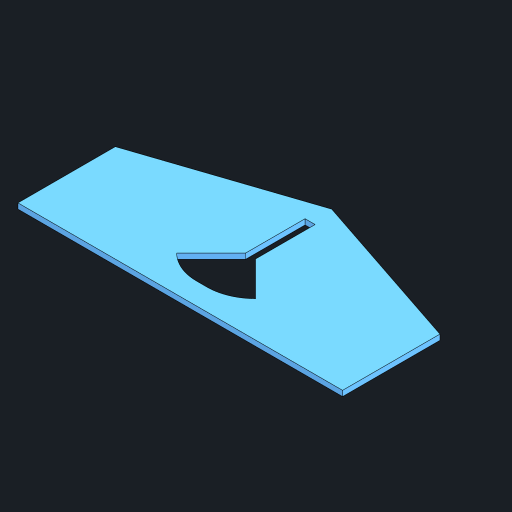
# Autodesk Inventor part: HoriWing
Saved by Autodesk Inventor 2023 (Build 270158000, 158)
## iProperties
Created: 2022-06-06
Part Number: HoriWing
Material: スタイロフォームIB
Document SubType Name: Modeling
Designer: neko2
Density: 0.027 g/cm^3
Appearance: スタイロフォームIB
Mass: 3.48774 g
Surface Area: 570.074 cm^2
Volume: 129.176 cm^3
Author: neko2
Autodesk Inventor part; units mm, degrees
ref_plane "YZ Plane" through (0, 0, 0) normal (1, 0, 0) x (0, 1, 0)
ref_plane "XZ Plane" through (0, 0, 0) normal (0, 1, 0) x (-1, 0, 0)
ref_plane "XY Plane" through (0, 0, 0) normal (0, 0, 1) x (1, 0, 0)
sketch "スケッチ1" plane through (0, 0, 0) normal (0, 1, 0) x (-1, 0, 0)
  line L0 (0, 0) -> (0, -342.0104)
  line L1 (0, -120) -> (-4.65, -120)
  line L2 (-4.65, -120) -> (-4.65, -65)
  line L3 (-150, -90) -> (0, -140)
  line L4 (0, 0) -> (-150, 0)
  line L5 (-150, 0) -> (-150, -90)
  line L6 (4.65, -120) -> (4.65, -65)
  line L7 (0, -120) -> (4.65, -120)
  line L8 (64.65, 0) -> (64.65, 0)
  line L9 (150, -90) -> (0, -140)
  line L10 (0, 0) -> (150, 0)
  line L11 (150, 0) -> (150, -90)
  line L12 (0, -70.9027) -> (0, -15.9027) construction
  arc A0 (-4.65, -20) -> (-36.4698, -33.1802) centre (-4.65, -65) ccw
  line L13 (-4.65, -65) -> (-36.4698, -33.1802) construction
  line L14 (-4.65, -65) -> (-4.65, -20) construction
  line L15 (-36.4698, -33.1802) -> (-4.65, -65)
  line L16 (-4.65, -20) -> (0, -20)
  arc A1 (36.4698, -33.1802) -> (4.65, -20) centre (4.65, -65) ccw
  line L17 (4.65, -65) -> (36.4698, -33.1802) construction
  line L18 (36.4698, -33.1802) -> (4.65, -65)
  line L19 (4.65, -20) -> (0, -20)
  line L20 (-150, -40) -> (-70, -40)
  line L21 (-70, -40) -> (-70, 0)
  line L22 (150, -40) -> (70, -40)
  line L23 (70, -40) -> (70, 0)
  point P0 (-4.65, -65)
  point P1 (4.65, -65)
  point P2 (70, 0)
  dimension "d0" = 9.3
  dimension "d3" = 300
  dimension "d5" = 140
  dimension "d6" = 50
  dimension "d13" = 55
  dimension "d14" = 20
  dimension "d20" = 45
  dimension "d21" = 45
  dimension "d22" = 40
  dimension "d23" = 80
  constraints: 48 end point, 10 symmetric about line, 7 point on line, 4 perpendicular, 4 point on circle, 3 horizontal, 2 centre point, 2 vertical, 1 coincident, 1 collinear, 1 other
  measures "d0" diameter of L2 L0
  measures "d3" diameter of L4.end L0
  measures "d5" distance of L0.start L3.end
  measures "d6" vertical distance of L3.start L3.end
  measures "d13" distance of L6.start L6.end
  measures "d14" distance of L3.end L1.start
  measures "d20" radius of A0
  measures "d21" angle of L14 L13
  measures "d22" distance of L20.end L21.end
  measures "d23" distance of L20.start L20.end
extrude "押し出し1" add sketch "スケッチ1" along normal blind 5 contours L10 L23 L22 L11 L9 L0 L7 L6 L18 A1 L19 | L0 L16 A0 L15 L2 L1 L3 L5 L20 L21 L4 | L21 L20 L5 L4 | L10 L11 L22 L23
